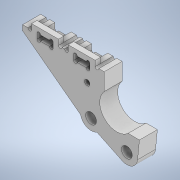
# Autodesk Inventor part: 後ろウィング固定フレーム中詰め
Saved by Autodesk Inventor 2020.2 (Build 242310000, 310)
## iProperties
Created: 2020-05-06
Part Number: 後ろウィング固定フレーム中詰め
Material: 一般
Document SubType Name: Modeling
Designer: mozar
Density: 1 g/cm^3
Appearance: 既定
Author: mozar
Autodesk Inventor part; units mm, degrees
ref_plane "YZ Plane" through (0, 0, 0) normal (1, 0, 0) x (0, 1, 0)
ref_plane "XZ Plane" through (0, 0, 0) normal (0, 1, 0) x (-1, 0, 0)
ref_plane "XY Plane" through (0, 0, 0) normal (0, 0, 1) x (1, 0, 0)
sketch "スケッチ1" plane through (0, 0, 0) normal (0, 0, 1) x (1, 0, 0)
  circle A0 centre (111.885, -19) radius 1.5
  line L0 (89.885, -6) -> (94.885, -6)
  arc A1 (94.885, -6) -> (96.885, -6) centre (95.885, -6) ccw
  line L1 (96.885, -6) -> (96.885, -3)
  arc A2 (96.885, -3) -> (94.885, -3) centre (95.885, -3) ccw
  line L2 (94.885, -3) -> (89.885, -3)
  arc A3 (89.885, -3) -> (87.885, -3) centre (88.885, -3) ccw
  line L3 (87.885, -3) -> (87.885, -6)
  arc A4 (87.885, -6) -> (89.885, -6) centre (88.885, -6) ccw
  arc A5 (76.4397, -3) -> (74.4397, -3) centre (75.4397, -3) ccw
  line L4 (74.4397, -3) -> (69.4397, -3)
  arc A6 (69.4397, -3) -> (67.4397, -3) centre (68.4397, -3) ccw
  line L5 (67.4397, -3) -> (67.4397, -6)
  arc A7 (67.4397, -6) -> (69.4397, -6) centre (68.4397, -6) ccw
  line L6 (69.4397, -6) -> (74.4397, -6)
  arc A8 (74.4397, -6) -> (76.4397, -6) centre (75.4397, -6) ccw
  line L7 (76.4397, -6) -> (76.4397, -3)
  line L8 (64.4397, -3) -> (64.4397, 0)
  line L9 (64.4397, 0) -> (79.4397, 0)
  line L10 (79.4397, 0) -> (79.4397, -3)
  arc A9 (79.4397, -3) -> (81.4397, -3) centre (80.4397, -3) ccw
  line L11 (81.4397, -3) -> (82.885, -3)
  arc A10 (82.885, -3) -> (84.885, -3) centre (83.885, -3) ccw
  line L12 (84.885, -3) -> (84.885, 0)
  line L13 (84.885, 0) -> (99.885, 0)
  line L14 (99.885, 0) -> (99.885, -3)
  arc A11 (99.885, -3) -> (101.885, -3) centre (100.885, -3) ccw
  line L15 (101.885, -3) -> (104.8897, -3)
  line L16 (104.8897, -3) -> (116.6369, -13.86)
  arc A12 (108.6424, -25.2037) -> (116.6369, -13.86) centre (111.885, -19) ccw
  arc A13 (108.5771, -25.2225) -> (108.6424, -25.2037) centre (95.0604, 21.7941) ccw
  line L17 (108.5771, -25.2225) -> (69.3788, -9.8882)
  arc A14 (65.1115, -8.2188) -> (69.3788, -9.8882) centre (68.4397, -6) ccw
  line L18 (65.1115, -8.2188) -> (59.4397, -6)
  line L19 (59.4397, -6) -> (59.4397, -3)
  line L20 (59.4397, -3) -> (62.4397, -3)
  arc A15 (62.4397, -3) -> (64.4397, -3) centre (63.4397, -3) ccw
  circle A16 centre (111.885, -19) radius 9
  circle A17 centre (111.885, -19) radius 9.5
  line L21 (111.8011, -25.9995) -> (171.7968, -26.719)
  circle A18 centre (111.885, -19) radius 14.5
  line L22 (111.7412, -30.9991) -> (171.7368, -31.7186)
  line L23 (93.2393, -9) -> (91.5308, -9)
  arc A19 (84.885, -6) -> (91.5308, -9) centre (88.885, -6) ccw
  line L24 (84.885, -6) -> (84.885, -3)
  arc A20 (91.5308, 0) -> (84.885, -3) centre (88.885, -3) ccw
  line L25 (91.5308, 0) -> (93.2393, 0)
  arc A21 (99.885, -3) -> (93.2393, 0) centre (95.885, -3) ccw
  line L26 (99.885, -3) -> (99.885, -6)
  arc A22 (93.2393, -9) -> (99.885, -6) centre (95.885, -6) ccw
  line L27 (72.7939, -9) -> (71.0854, -9)
  arc A23 (64.4397, -6) -> (71.0854, -9) centre (68.4397, -6) ccw
  line L28 (64.4397, -6) -> (64.4397, -3)
  arc A24 (71.0854, 0) -> (64.4397, -3) centre (68.4397, -3) ccw
  line L29 (71.0854, 0) -> (72.7939, 0)
  arc A25 (79.4397, -3) -> (72.7939, 0) centre (75.4397, -3) ccw
  line L30 (79.4397, -3) -> (79.4397, -6)
  arc A26 (72.7939, -9) -> (79.4397, -6) centre (75.4397, -6) ccw
  line L31 (69.2325, -6.6095) -> (108.7075, -22.0521)
  arc A27 (108.7075, -22.0521) -> (109.1445, -21.9137) centre (95.0604, 21.7941) ccw
  arc A28 (109.1445, -21.9137) -> (114.6004, -16.0628) centre (111.885, -19) ccw
  line L32 (114.6004, -16.0628) -> (103.7154, -6)
  line L33 (103.7154, -6) -> (103.5308, -6)
  arc A29 (96.885, -3) -> (103.5308, -6) centre (100.885, -3) ccw
  line L34 (96.885, -3) -> (87.885, -3)
  arc A30 (82.1624, -6.61) -> (87.885, -3) centre (83.885, -3) ccw
  arc A31 (76.4397, -3) -> (82.1624, -6.61) centre (80.4397, -3) ccw
  line L35 (76.4397, -3) -> (67.4397, -3)
  arc A32 (66.5221, -5.5493) -> (67.4397, -3) centre (63.4397, -3) ccw
  line L36 (66.5221, -5.5493) -> (67.4438, -5.9098)
  arc A33 (67.4438, -5.9098) -> (69.2325, -6.6095) centre (68.4397, -6) ccw
  circle A34 centre (111.885, -19) radius 1.5
  line L37 (111.885, -19) -> (111.885, 12.5174) construction
  line L38 (118.885, -19) -> (118.885, 12.5174)
  line L39 (104.885, 12.5174) -> (104.885, -19)
  arc A35 (104.885, -19) -> (118.885, -19) centre (111.885, -19) ccw
  arc A36 (118.885, 12.5174) -> (104.885, 12.5174) centre (111.885, 12.5174) ccw
  circle A37 centre (95.4507, -12.9865) radius 3
  circle A38 centre (121.1072, -35.6118) radius 4.5
  circle A39 centre (71.9397, -13.746) radius 4.5
  line L40 (118.9115, -39.5397) -> (104.8098, -31.6566)
  line L41 (106.4851, -32.457) -> (70.2638, -17.9223)
  line L42 (125.2948, -33.9642) -> (118.399, -16.4372)
  arc A40 (108.6424, -25.2037) -> (116.6369, -13.86) centre (111.885, -19) ccw
  point P0 (0, 0)
  point P1 (0, 0)
  point P2 (111.885, -3.2413)
  point P3 (69.5283, -9.9466)
  point P4 (118.885, -17.6725)
  point P5 (118.399, -16.4372)
  point P6 (123.0482, -28.2539)
  point P7 (105.6218, -32.1106)
  point P8 (97.5091, -20.8927)
  point P9 (107.3125, -5.2398)
  point P10 (104.885, -6.3016)
  point P11 (104.885, -3)
  dimension "d10" = 9
  dimension "d0" = 18
  dimension "d1" = 0.5
  dimension "d2" = 5
  dimension "d3" = 5
  dimension "d4" = 3
  dimension "d5" = 3
  dimension "d6" = 3
  dimension "d7" = 14
  dimension "d8" = 6
  dimension "d9" = 9
  constraints: 88 end point, 71 point on circle, 40 centre point, 13 tangent, 2 parallel, 1 coincident, 1 midpoint, 1 vertical, 33 other
  measures "d0" diameter of A16
  measures "d1" radial gap between concentric circles of A16 A17
  measures "d2" radial gap between concentric circles of A17 A18
  measures "d3" distance between parallel lines of L21 L22
  measures "d4" distance between parallel lines of L0 L23
  measures "d5" distance between parallel lines of L6 L27
  measures "d6" distance between parallel lines of L17 L31
  measures "d7" diameter of A36
  measures "d8" diameter of A37
  measures "d9" diameter of A38
sketch "スケッチ2" plane through (0, 0, 0) normal (0, 0, 1) x (1, 0, 0)
  circle A0 centre (111.885, -19) radius 9.5 projected
  circle A1 centre (111.885, -19) radius 14.5 projected
  circle A2 centre (117.5177, -35.5687) radius 4.5
  circle A3 centre (71.9397, -13.746) radius 4.5 projected
  circle A4 centre (95.4507, -12.9865) radius 3 projected
  arc A5 (96.885, -3) -> (103.5308, -6) centre (100.885, -3) ccw projected
  line L0 (101.885, -3) -> (104.8897, -3) projected
  line L1 (59.4397, -3) -> (62.4397, -3) projected
  line L2 (59.4397, -6) -> (59.4397, -3) projected
  arc A6 (94.885, -6) -> (96.885, -6) centre (95.885, -6) ccw projected
  line L3 (96.885, -6) -> (96.885, -3) projected
  arc A7 (96.885, -3) -> (94.885, -3) centre (95.885, -3) ccw projected
  arc A8 (89.885, -3) -> (87.885, -3) centre (88.885, -3) ccw projected
  line L4 (87.885, -3) -> (87.885, -6) projected
  arc A9 (87.885, -6) -> (89.885, -6) centre (88.885, -6) ccw projected
  line L5 (89.885, -6) -> (94.885, -6) projected
  line L6 (94.885, -3) -> (89.885, -3) projected
  arc A10 (76.4397, -3) -> (74.4397, -3) centre (75.4397, -3) ccw projected
  line L7 (74.4397, -3) -> (69.4397, -3) projected
  arc A11 (69.4397, -3) -> (67.4397, -3) centre (68.4397, -3) ccw projected
  line L8 (67.4397, -3) -> (67.4397, -6) projected
  arc A12 (67.4438, -5.9098) -> (69.2325, -6.6095) centre (68.4397, -6) ccw projected
  line L9 (69.4397, -6) -> (74.4397, -6) projected
  arc A13 (74.4397, -6) -> (76.4397, -6) centre (75.4397, -6) ccw projected
  line L10 (76.4397, -6) -> (76.4397, -3) projected
  line L11 (111.7412, -30.9991) -> (171.7368, -31.7186) projected
  line L12 (111.8011, -25.9995) -> (171.7968, -26.719) projected
  circle A14 centre (117.5177, -35.5687) radius 3
  circle A15 centre (71.9397, -13.746) radius 3
  circle A16 centre (117.5177, -35.5687) radius 6
  circle A17 centre (95.4507, -12.9865) radius 6
  circle A18 centre (71.9397, -13.746) radius 6
  line L13 (111.885, -19) -> (111.885, 24.2673) construction
  line L14 (118.885, -19) -> (118.885, 24.2673)
  line L15 (104.885, 24.2673) -> (104.885, -19)
  arc A19 (104.885, -19) -> (118.885, -19) centre (111.885, -19) ccw
  arc A20 (118.885, 24.2673) -> (104.885, 24.2673) centre (111.885, 24.2673) ccw
  line L16 (123.4874, -36.1712) -> (124.4986, -26.1518)
  line L17 (101.885, -3) -> (62.4397, -3)
  line L18 (59.4397, -6) -> (66.9734, -17.1128)
  line L19 (114.9266, -40.9804) -> (69.3486, -19.1576)
  arc A21 (69.2325, -6.6095) -> (69.4397, -6) centre (68.4397, -6) ccw
  point P0 (0, 0)
  point P1 (111.885, 2.6337)
  point P2 (118.2233, -26.0765)
  point P3 (104.885, -12.5774)
  point P4 (104.885, -3)
  point P5 (87.885, -3)
  point P6 (76.4397, -3)
  point P7 (67.4397, -3)
  dimension "d11" = 6
  dimension "d12" = 6
  dimension "d13" = 3
  dimension "d14" = 3
  dimension "d15" = 3
  dimension "d16" = 14
  dimension "d52" = 9
  constraints: 16 end point, 10 point on circle, 9 centre point, 9 tangent, 3 coincident, 1 horizontal, 1 midpoint, 1 parallel, 1 point on line, 1 vertical, 3 other
  measures "d11" diameter of A14
  measures "d12" diameter of A15
  measures "d13" radial gap between concentric circles of A14 A16
  measures "d14" radial gap between concentric circles of A4 A17
  measures "d15" radial gap between concentric circles of A15 A18
  measures "d16" diameter of A20
  measures "d52" diameter of A2
extrude "押し出し1" add sketch "スケッチ2" against normal blind 10 contours L12 A1 A16 A17 L15 A0 | L16 L11 A16 A1 | A1 A17 A6 L3 L17 L0 L15 | A16 L11 A1 | A1 L11 A16 | L16 A16 L11 | A17 A1 | A4 | A1 A17 | L11 A16 A1 A2 | A1 A2 L11 | L11 A2 A1 A16 | A17 A1 A16 L19 A18 L18 L2 L1 L17 L8 A12 A21 L9 A13 L10 L4 A9 L5 A6 | A14 | A2 A1 | A1 A2 | A18 | A3 | A15
hole "穴1" at (71.9397, -13.746, 0) at (95.4507, -12.9865, 0) at (117.5177, -35.5687, 0) direction (0, 0, -1) diameter 6 depth 12 tip angle 118
sketch "スケッチ3" plane through (0, 0, 0) normal (0, 0, 1) x (1, 0, 0)
  line L0 (-101.5, 48) -> (108.5, 48)
  circle A0 centre (111.885, -19) radius 4
  circle A1 centre (171.8807, -19.7195) radius 4
  circle A2 centre (111.885, -19) radius 7
  circle A3 centre (171.8807, -19.7195) radius 7
  line L1 (171.8807, -19.7195) -> (111.885, -19) construction
  line L2 (171.9647, -12.72) -> (111.969, -12.0005)
  line L3 (111.8011, -25.9995) -> (171.7968, -26.719)
  arc A4 (171.7968, -26.719) -> (171.9647, -12.72) centre (171.8807, -19.7195) ccw
  arc A5 (111.969, -12.0005) -> (111.8011, -25.9995) centre (111.885, -19) ccw
  line L4 (173.7961, -12.9866) -> (250.1906, -34.7195)
  circle A6 centre (241.9819, -63.5746) radius 30
  line L5 (268.18, -78.1916) -> (221.9512, -41.2414)
  line L6 (221.9512, -41.2414) -> (169.9654, -26.4523)
  line L7 (271.9819, -113.1361) -> (271.9819, -54.8199)
  line L8 (111.885, -19) -> (111.885, 41) construction
  line L9 (118.885, -19) -> (118.885, 41)
  line L10 (104.885, 41) -> (104.885, -19)
  arc A7 (104.885, -19) -> (118.885, -19) centre (111.885, -19) ccw
  arc A8 (118.885, 41) -> (104.885, 41) centre (111.885, 41) ccw
  circle A9 centre (29.4318, 47.238) radius 30
  line L11 (113.3193, 34.1485) -> (35.5787, 17.8745)
  line L12 (-0.5585, 48) -> (57.5489, 36.7771)
  line L13 (57.5489, 36.7771) -> (110.4508, 47.8515)
  circle A10 centre (113.5, -20) radius 68
  line L14 (321.9635, -82.9551) -> (60.2705, 100.2843)
  line L15 (259.1892, -39) -> (111.885, -19)
  arc A11 (93.5924, -27.1048) -> (135.371, -5.9244) centre (95.0604, 21.7941) ccw
  arc A12 (135.371, -5.9244) -> (135.8476, -3.6716) centre (132.899, -4.2246) ccw
  arc A13 (135.8476, -3.6716) -> (83.1833, 18.5565) centre (102.1579, -9.9896) ccw
  line L16 (111.885, -19) -> (112.6892, 40.9946) construction
  line L17 (118.8844, -19.0938) -> (119.6886, 40.9008)
  line L18 (105.6898, 41.0884) -> (104.8857, -18.9062)
  arc A14 (104.8857, -18.9062) -> (118.8844, -19.0938) centre (111.885, -19) ccw
  arc A15 (119.6886, 40.9008) -> (105.6898, 41.0884) centre (112.6892, 40.9946) ccw
  line L19 (164.9949, 48) -> (164.9949, 26)
  line L20 (164.9949, 26) -> (327.4949, -102)
  circle A16 centre (116.2926, -40) radius 68
  circle A17 centre (-98.885, 0) radius 67.5
  line L21 (321.3633, -8.501) -> (-152.6681, 78.4982)
  line L22 (104.8897, -3) -> (104.8897, 0)
  line L23 (104.8897, -3) -> (72.0656, -3)
  line L24 (72.0656, 0) -> (104.8897, 0)
  circle A18 centre (83.3769, -17.5) radius 13.85
  point P0 (0, 0)
  point P1 (141.8829, -19.3597)
  point P2 (111.885, 11)
  point P3 (105.885, 0)
  point P4 (105.885, 0)
  point P5 (23.7328, -42.729)
  point P6 (112.2871, 10.9973)
  dimension "d26" = 8
  dimension "d27" = 8
  dimension "d28" = 3
  dimension "d29" = 3
  dimension "d30" = 60
  dimension "d31" = 14
  dimension "d32" = 14
  dimension "d33" = 60
  dimension "d34" = 14
  dimension "d35" = 60
  dimension "d36" = 14
  dimension "d37" = 6
  dimension "d38" = 35
  dimension "d39" = 13.271
  dimension "d40" = 14
  dimension "d41" = 20
  dimension "d42" = 15
  dimension "d43" = 22
  dimension "d44" = 150
  dimension "d45" = 162.5
  dimension "d46" = 0
  dimension "d47" = 136
  dimension "d48" = 136
  dimension "d49" = 135
  dimension "d50" = 38.227
  dimension "d51" = 18
  constraints: 56 end point, 28 point on circle, 25 tangent, 18 centre point, 4 equal length, 3 coincident, 3 horizontal, 3 midpoint, 3 parallel, 3 vertical, 2 point on line, 1 concentric, 15 other
  measures "d26" diameter of A0
  measures "d27" diameter of A1
  measures "d28" radial gap between concentric circles of A0 A2
  measures "d30" distance of L1.start L1.end
  measures "d31" diameter of A5
  measures "d32" distance from line of L4 L5.end
  measures "d33" diameter of A6
  measures "d34" diameter of A8
  measures "d35" diameter of A9
  measures "d36" distance from line of L11 L12.end
  measures "d37" horizontal distance of L1.end point (105.885, 0)
  measures "d38" angle of L14 L0
  measures "d40" diameter of A15
  measures "d41" vertical distance of L15.start L1.end
  measures "d42" vertical distance of L1.start L4.end
  measures "d43" distance of L19.start L19.end
  measures "d44" vertical distance of L19.start L20.end
  measures "d45" distance from line of L19 L20.end
  measures "d46" distance from line of L19.start L0
  measures "d47" diameter of A10
  measures "d48" diameter of A16
  measures "d49" diameter of A17
  measures "d50" angle of L0 L20
  measures "d51" distance from line of L5.start L20
sketch "スケッチ4" plane through (0, 0, 0) normal (0, 0, 1) x (1, 0, 0)
  circle A0 centre (117.5177, -35.5687) radius 1.5
  circle A1 centre (95.4507, -12.9865) radius 1.5
  circle A2 centre (97.5945, -29.101) radius 1.5
  circle A3 centre (111.885, -19) radius 1.5
  line L0 (116.6369, -13.86) -> (104.8897, -3)
  line L1 (104.8897, -3) -> (101.885, -3)
  arc A4 (99.885, -3) -> (101.885, -3) centre (100.885, -3) ccw
  line L2 (99.885, -3) -> (99.885, 0)
  line L3 (99.885, 0) -> (84.885, 0)
  line L4 (84.885, 0) -> (84.885, -3)
  arc A5 (82.885, -3) -> (84.885, -3) centre (83.885, -3) ccw
  line L5 (82.885, -3) -> (81.4397, -3)
  arc A6 (79.4397, -3) -> (81.4397, -3) centre (80.4397, -3) ccw
  line L6 (79.4397, -3) -> (79.4397, 0)
  line L7 (79.4397, 0) -> (64.4397, 0)
  line L8 (64.4397, 0) -> (64.4397, -3)
  arc A7 (62.4397, -3) -> (64.4397, -3) centre (63.4397, -3) ccw
  line L9 (62.4397, -3) -> (59.4397, -3)
  line L10 (59.4397, -3) -> (59.4397, -6)
  line L11 (59.4397, -6) -> (65.1115, -8.2188)
  arc A8 (65.1115, -8.2188) -> (69.3788, -9.8882) centre (68.4397, -6) ccw
  line L12 (69.3788, -9.8882) -> (97.5091, -20.8927)
  arc A9 (97.5091, -20.8927) -> (98.5543, -24.7045) centre (111.885, -19) ccw
  arc A10 (98.5543, -24.7045) -> (97.6262, -33.6009) centre (97.5945, -29.101) ccw
  line L13 (97.6262, -33.6009) -> (107.1669, -33.5336)
  line L14 (107.1669, -33.5336) -> (114.849, -39.192)
  arc A11 (114.849, -39.192) -> (121.9415, -34.7438) centre (117.5177, -35.5687) ccw
  line L15 (121.9415, -34.7438) -> (118.7664, -17.7168)
  arc A12 (118.7664, -17.7168) -> (116.6369, -13.86) centre (111.885, -19) ccw
  line L16 (69.4397, -3) -> (74.4397, -3)
  arc A13 (76.4397, -3) -> (74.4397, -3) centre (75.4397, -3) ccw
  line L17 (76.4397, -3) -> (76.4397, -6)
  arc A14 (74.4397, -6) -> (76.4397, -6) centre (75.4397, -6) ccw
  line L18 (74.4397, -6) -> (69.4397, -6)
  arc A15 (67.4397, -6) -> (69.4397, -6) centre (68.4397, -6) ccw
  line L19 (67.4397, -6) -> (67.4397, -3)
  arc A16 (69.4397, -3) -> (67.4397, -3) centre (68.4397, -3) ccw
  arc A17 (94.885, -6) -> (96.885, -6) centre (95.885, -6) ccw
  line L20 (94.885, -6) -> (89.885, -6)
  arc A18 (87.885, -6) -> (89.885, -6) centre (88.885, -6) ccw
  line L21 (87.885, -6) -> (87.885, -3)
  arc A19 (89.885, -3) -> (87.885, -3) centre (88.885, -3) ccw
  line L22 (89.885, -3) -> (94.885, -3)
  arc A20 (96.885, -3) -> (94.885, -3) centre (95.885, -3) ccw
  line L23 (96.885, -3) -> (96.885, -6)
  circle A21 centre (95.4507, -12.9865) radius 3 projected
  circle A22 centre (71.9397, -13.746) radius 3 projected
  circle A23 centre (117.5177, -35.5687) radius 3 projected
  arc A24 (87.885, -6) -> (89.885, -6) centre (88.885, -6) ccw projected
  line L24 (87.885, -6) -> (87.885, -3) projected
  line L25 (87.885, -3) -> (76.4397, -3) projected
  line L26 (76.4397, -3) -> (76.4397, -6) projected
  arc A25 (74.4397, -6) -> (76.4397, -6) centre (75.4397, -6) ccw projected
  line L27 (74.4397, -6) -> (69.4397, -6) projected
  arc A26 (67.4397, -6) -> (69.4397, -6) centre (68.4397, -6) ccw projected
  line L28 (67.4397, -6) -> (67.4397, -3) projected
  line L29 (67.4397, -3) -> (59.4397, -3) projected
  line L30 (59.4397, -3) -> (59.4397, -6) projected
  line L31 (59.4397, -6) -> (66.9734, -17.1128) projected
  arc A27 (66.9734, -17.1128) -> (69.3486, -19.1576) centre (71.9397, -13.746) ccw projected
  line L32 (69.3486, -19.1576) -> (114.9266, -40.9804) projected
  arc A28 (114.9266, -40.9804) -> (123.4874, -36.1712) centre (117.5177, -35.5687) ccw projected
  line L33 (123.4874, -36.1712) -> (124.4986, -26.1518) projected
  line L34 (124.4986, -26.1518) -> (118.2233, -26.0765) projected
  arc A29 (104.885, -12.5774) -> (118.2233, -26.0765) centre (111.885, -19) ccw projected
  line L35 (104.885, -12.5774) -> (104.885, -3) projected
  line L36 (104.885, -3) -> (96.885, -3) projected
  line L37 (96.885, -3) -> (96.885, -6) projected
  arc A30 (94.885, -6) -> (96.885, -6) centre (95.885, -6) ccw projected
  line L38 (94.885, -6) -> (89.885, -6) projected
  point P0 (0, 0)
  point P1 (0, 0)
  point P2 (74.2011, -11.7746)
  point P3 (71.6162, -10.7635)
  point P4 (99.4867, -33.5878)
  point P5 (93.3734, -30.6607)
  constraints: 48 end point, 34 point on circle, 21 centre point, 9 horizontal, 9 vertical, 89 other
extrude "押し出し2" add sketch "スケッチ4" against normal blind 10 contours L13 A10 L32 | L12 A22 picked at (72.7177, -11.1035)
extrude "押し出し3" cut sketch "スケッチ4" against normal blind 10 contours L32 A27 L31 L11 A8 L12 A22 A9 A10
hole "穴2" at (97.5945, -29.101, 0) direction (0, 0, -1) diameter 3 depth 12 tip angle 118
extrude "押し出し4" add sketch "スケッチ4" against normal blind 10 contours A21
sketch "スケッチ5" plane through (0, 0, 0) normal (0, 0, 1) x (1, 0, 0)
  circle A0 centre (95.4507, -12.9865) radius 1.5 projected
  circle A1 centre (97.5945, -29.101) radius 1.5 projected
  arc A2 (98.5543, -24.7045) -> (97.6262, -33.6009) centre (97.5945, -29.101) ccw projected
  line L0 (97.6262, -33.6009) -> (99.4867, -33.5878) projected
  line L1 (99.4867, -33.5878) -> (114.9266, -40.9804) projected
  arc A3 (114.9266, -40.9804) -> (123.4874, -36.1712) centre (117.5177, -35.5687) ccw projected
  line L2 (123.4874, -36.1712) -> (124.4986, -26.1518) projected
  line L3 (124.4986, -26.1518) -> (118.2233, -26.0765) projected
  arc A4 (104.885, -12.5774) -> (118.2233, -26.0765) centre (111.885, -19) ccw projected
  line L4 (104.885, -12.5774) -> (104.885, -3) projected
  line L5 (104.885, -3) -> (96.885, -3) projected
  line L6 (96.885, -3) -> (96.885, -6) projected
  arc A5 (94.885, -6) -> (96.885, -6) centre (95.885, -6) ccw projected
  line L7 (94.885, -6) -> (89.885, -6) projected
  arc A6 (87.885, -6) -> (89.885, -6) centre (88.885, -6) ccw projected
  line L8 (87.885, -6) -> (87.885, -3) projected
  line L9 (87.885, -3) -> (76.4397, -3) projected
  line L10 (76.4397, -3) -> (76.4397, -6) projected
  arc A7 (74.4397, -6) -> (76.4397, -6) centre (75.4397, -6) ccw projected
  line L11 (74.4397, -6) -> (69.4397, -6) projected
  arc A8 (67.4397, -6) -> (69.4397, -6) centre (68.4397, -6) ccw projected
  line L12 (67.4397, -6) -> (67.4397, -3) projected
  line L13 (67.4397, -3) -> (59.4397, -3) projected
  line L14 (59.4397, -3) -> (59.4397, -6) projected
  line L15 (59.4397, -6) -> (65.1115, -8.2188) projected
  arc A9 (65.1115, -8.2188) -> (69.3788, -9.8882) centre (68.4397, -6) ccw projected
  line L16 (69.3788, -9.8882) -> (97.5091, -20.8927) projected
  arc A10 (97.5091, -20.8927) -> (98.5543, -24.7045) centre (111.885, -19) ccw projected
  line L17 (96.885, -3) -> (104.885, -3) projected
  line L18 (99.885, -3) -> (84.885, -3)
  line L19 (84.885, -3) -> (84.885, 0)
  line L20 (84.885, 0) -> (99.885, 0)
  line L21 (99.885, 0) -> (99.885, -3)
  line L22 (76.4397, -3) -> (87.885, -3) projected
  line L23 (79.4397, -3) -> (64.4397, -3)
  line L24 (64.4397, -3) -> (64.4397, 0)
  line L25 (64.4397, 0) -> (79.4397, 0)
  line L26 (79.4397, 0) -> (79.4397, -3)
  circle A11 centre (95.885, -3) radius 1
  circle A12 centre (88.885, -3) radius 1
  circle A13 centre (75.4397, -3) radius 1
  circle A14 centre (68.4397, -3) radius 1
  line L27 (96.885, -3) -> (96.885, -6) projected
  line L28 (87.885, -6) -> (87.885, -3) projected
  line L29 (67.4397, -6) -> (67.4397, -3) projected
  point P0 (0, 0)
  point P1 (69.4397, -3)
  point P2 (74.4397, -3)
  point P3 (89.885, -3)
  point P4 (94.885, -3)
  dimension "d66" = 15
  dimension "d67" = 3
  dimension "d68" = 15
  dimension "d69" = 3
  dimension "d70" = 3
  dimension "d71" = 3
  dimension "d72" = 2
  dimension "d73" = 2
  dimension "d74" = 2
  dimension "d75" = 2
  constraints: 16 end point, 6 point on line, 4 centre point, 4 parallel, 4 tangent, 2 horizontal, 2 perpendicular
  measures "d66" distance of L19.end L20.end
  measures "d67" distance of L18.end L19.end
  measures "d68" distance of L24.end L25.end
  measures "d69" distance of L23.end L24.end
  measures "d70" distance between parallel lines of L19 L8
  measures "d71" distance between parallel lines of L26 L10
  measures "d72" diameter of A11
  measures "d73" diameter of A12
  measures "d74" diameter of A13
  measures "d75" diameter of A14
extrude "押し出し5" add sketch "スケッチ5" against normal blind 3 contours L24 L25 L26 L9 A13 L23 A14 L13 | L5 A11 L18 A12 L9 L19 L20 L21
sketch "スケッチ6" plane through (0, 0, 0) normal (0, 0, 1) x (1, 0, 0)
  line L0 (64.4397, -3) -> (59.4397, -3) projected
  line L1 (59.4397, -3) -> (59.4397, -6) projected
  line L2 (59.4397, -6) -> (65.1115, -8.2188) projected
  arc A0 (65.1115, -8.2188) -> (69.3788, -9.8882) centre (68.4397, -6) ccw projected
  line L3 (69.3788, -9.8882) -> (97.5091, -20.8927) projected
  arc A1 (97.5091, -20.8927) -> (98.5543, -24.7045) centre (111.885, -19) ccw projected
  arc A2 (98.5543, -24.7045) -> (97.6262, -33.6009) centre (97.5945, -29.101) ccw projected
  line L4 (97.6262, -33.6009) -> (99.4867, -33.5878) projected
  line L5 (99.4867, -33.5878) -> (114.9266, -40.9804) projected
  arc A3 (114.9266, -40.9804) -> (123.4874, -36.1712) centre (117.5177, -35.5687) ccw projected
  line L6 (123.4874, -36.1712) -> (124.4986, -26.1518) projected
  line L7 (124.4986, -26.1518) -> (118.2233, -26.0765) projected
  arc A4 (104.885, -12.5774) -> (118.2233, -26.0765) centre (111.885, -19) ccw projected
  line L8 (104.885, -12.5774) -> (104.885, -3) projected
  line L9 (104.885, -3) -> (99.885, -3) projected
  line L10 (99.885, -3) -> (99.885, 0) projected
  line L11 (99.885, 0) -> (84.885, 0) projected
  line L12 (84.885, 0) -> (84.885, -3) projected
  line L13 (84.885, -3) -> (79.4397, -3) projected
  line L14 (79.4397, -3) -> (79.4397, 0) projected
  line L15 (79.4397, 0) -> (64.4397, 0) projected
  line L16 (64.4397, 0) -> (64.4397, -3) projected
  arc A5 (69.4397, -3) -> (67.4397, -3) centre (68.4397, -3) ccw projected
  line L17 (69.4397, -3) -> (74.4397, -3) projected
  arc A6 (76.4397, -3) -> (74.4397, -3) centre (75.4397, -3) ccw projected
  line L18 (76.4397, -3) -> (76.4397, -6) projected
  arc A7 (74.4397, -6) -> (76.4397, -6) centre (75.4397, -6) ccw projected
  line L19 (74.4397, -6) -> (69.4397, -6) projected
  arc A8 (67.4397, -6) -> (69.4397, -6) centre (68.4397, -6) ccw projected
  line L20 (67.4397, -6) -> (67.4397, -3) projected
  circle A9 centre (95.4507, -12.9865) radius 1.5 projected
  circle A10 centre (97.5945, -29.101) radius 1.5 projected
  arc A11 (89.885, -3) -> (87.885, -3) centre (88.885, -3) ccw projected
  line L21 (89.885, -3) -> (94.885, -3) projected
  arc A12 (96.885, -3) -> (94.885, -3) centre (95.885, -3) ccw projected
  line L22 (96.885, -3) -> (96.885, -6) projected
  arc A13 (94.885, -6) -> (96.885, -6) centre (95.885, -6) ccw projected
  line L23 (94.885, -6) -> (89.885, -6) projected
  arc A14 (87.885, -6) -> (89.885, -6) centre (88.885, -6) ccw projected
  line L24 (87.885, -6) -> (87.885, -3) projected
  line L25 (99.885, -3) -> (104.885, -3) projected
  circle A15 centre (100.885, -3) radius 1
  line L26 (79.4397, -3) -> (84.885, -3) projected
  circle A16 centre (83.885, -3) radius 1
  circle A17 centre (80.4397, -3) radius 1
  line L27 (59.4397, -3) -> (64.4397, -3) projected
  circle A18 centre (63.4397, -3) radius 1
  line L28 (99.885, -3) -> (99.885, 0) projected
  line L29 (84.885, 0) -> (84.885, -3) projected
  line L30 (79.4397, -3) -> (79.4397, 0) projected
  point P0 (0, 0)
  dimension "d78" = 2
  dimension "d79" = 2
  dimension "d80" = 2
  dimension "d81" = 2
  constraints: 4 centre point, 4 point on line, 4 tangent
  measures "d78" diameter of A15
  measures "d79" diameter of A16
  measures "d80" diameter of A17
  measures "d81" diameter of A18
extrude "押し出し6" cut sketch "スケッチ6" against normal blind 10 contours A18 L0 | L0 A18 | A17 L13 | L13 A17 | A16 L13 | L13 A16 | A15 L9 | L9 A15
sketch "スケッチ7" plane through (0, 0, 0) normal (0, 0, 1) x (1, 0, 0)
  arc A0 (79.4397, -3) -> (81.4397, -3) centre (80.4397, -3) ccw projected
  line L0 (79.4397, -3) -> (79.4397, 0) projected
  line L1 (79.4397, 0) -> (64.4397, 0) projected
  line L2 (64.4397, 0) -> (64.4397, -3) projected
  arc A1 (62.4397, -3) -> (64.4397, -3) centre (63.4397, -3) ccw projected
  line L3 (62.4397, -3) -> (59.4397, -3) projected
  line L4 (59.4397, -3) -> (59.4397, -6) projected
  line L5 (59.4397, -6) -> (65.1115, -8.2188) projected
  arc A2 (65.1115, -8.2188) -> (69.3788, -9.8882) centre (68.4397, -6) ccw projected
  line L6 (69.3788, -9.8882) -> (97.5091, -20.8927) projected
  arc A3 (97.5091, -20.8927) -> (98.5543, -24.7045) centre (111.885, -19) ccw projected
  arc A4 (98.5543, -24.7045) -> (97.6262, -33.6009) centre (97.5945, -29.101) ccw projected
  line L7 (97.6262, -33.6009) -> (99.4867, -33.5878) projected
  line L8 (99.4867, -33.5878) -> (114.9266, -40.9804) projected
  arc A5 (114.9266, -40.9804) -> (123.4874, -36.1712) centre (117.5177, -35.5687) ccw projected
  line L9 (123.4874, -36.1712) -> (124.4986, -26.1518) projected
  line L10 (124.4986, -26.1518) -> (118.2233, -26.0765) projected
  arc A6 (104.885, -12.5774) -> (118.2233, -26.0765) centre (111.885, -19) ccw projected
  line L11 (104.885, -12.5774) -> (104.885, -3) projected
  line L12 (104.885, -3) -> (101.885, -3) projected
  arc A7 (99.885, -3) -> (101.885, -3) centre (100.885, -3) ccw projected
  line L13 (99.885, -3) -> (99.885, 0) projected
  line L14 (99.885, 0) -> (84.885, 0) projected
  line L15 (84.885, 0) -> (84.885, -3) projected
  arc A8 (82.885, -3) -> (84.885, -3) centre (83.885, -3) ccw projected
  line L16 (82.885, -3) -> (81.4397, -3) projected
  arc A9 (69.4397, -3) -> (67.4397, -3) centre (68.4397, -3) ccw projected
  line L17 (69.4397, -3) -> (74.4397, -3) projected
  arc A10 (76.4397, -3) -> (74.4397, -3) centre (75.4397, -3) ccw projected
  line L18 (76.4397, -3) -> (76.4397, -6) projected
  arc A11 (74.4397, -6) -> (76.4397, -6) centre (75.4397, -6) ccw projected
  line L19 (74.4397, -6) -> (69.4397, -6) projected
  arc A12 (67.4397, -6) -> (69.4397, -6) centre (68.4397, -6) ccw projected
  line L20 (67.4397, -6) -> (67.4397, -3) projected
  circle A13 centre (95.4507, -12.9865) radius 1.5 projected
  circle A14 centre (97.5945, -29.101) radius 1.5 projected
  arc A15 (89.885, -3) -> (87.885, -3) centre (88.885, -3) ccw projected
  line L21 (89.885, -3) -> (94.885, -3) projected
  arc A16 (96.885, -3) -> (94.885, -3) centre (95.885, -3) ccw projected
  line L22 (96.885, -3) -> (96.885, -6) projected
  arc A17 (94.885, -6) -> (96.885, -6) centre (95.885, -6) ccw projected
  line L23 (94.885, -6) -> (89.885, -6) projected
  arc A18 (87.885, -6) -> (89.885, -6) centre (88.885, -6) ccw projected
  line L24 (87.885, -6) -> (87.885, -3) projected
  arc A19 (98.5543, -24.7045) -> (97.6262, -33.6009) centre (97.5945, -29.101) ccw projected
  line L25 (59.4397, -3) -> (59.4397, -6) projected
  line L26 (94.8874, -32.6956) -> (59.4397, -6)
  arc A20 (98.5543, -24.7045) -> (97.6262, -33.6009) centre (97.5945, -29.101) ccw projected
  point P0 (0, 0)
  constraints: 2 end point, 1 point on circle, 1 tangent
extrude "押し出し7" add sketch "スケッチ7" against normal blind 10 contours L5 A2 L6 A3 A4 L26
sketch "スケッチ8" plane through (0, 0, 0) normal (0, 0, 1) x (1, 0, 0)
  arc A0 (79.4397, -3) -> (81.4397, -3) centre (80.4397, -3) ccw projected
  line L0 (79.4397, -3) -> (79.4397, 0) projected
  line L1 (79.4397, 0) -> (64.4397, 0) projected
  line L2 (64.4397, 0) -> (64.4397, -3) projected
  arc A1 (62.4397, -3) -> (64.4397, -3) centre (63.4397, -3) ccw projected
  line L3 (62.4397, -3) -> (59.4397, -3) projected
  line L4 (59.4397, -3) -> (59.4397, -6) projected
  line L5 (59.4397, -6) -> (94.8874, -32.6956) projected
  arc A2 (94.8874, -32.6956) -> (97.6262, -33.6009) centre (97.5945, -29.101) ccw projected
  line L6 (97.6262, -33.6009) -> (99.4867, -33.5878) projected
  line L7 (99.4867, -33.5878) -> (114.9266, -40.9804) projected
  arc A3 (114.9266, -40.9804) -> (123.4874, -36.1712) centre (117.5177, -35.5687) ccw projected
  line L8 (123.4874, -36.1712) -> (124.4986, -26.1518) projected
  line L9 (124.4986, -26.1518) -> (118.2233, -26.0765) projected
  arc A4 (104.885, -12.5774) -> (118.2233, -26.0765) centre (111.885, -19) ccw projected
  line L10 (104.885, -12.5774) -> (104.885, -3) projected
  line L11 (104.885, -3) -> (101.885, -3) projected
  arc A5 (99.885, -3) -> (101.885, -3) centre (100.885, -3) ccw projected
  line L12 (99.885, -3) -> (99.885, 0) projected
  line L13 (99.885, 0) -> (84.885, 0) projected
  line L14 (84.885, 0) -> (84.885, -3) projected
  arc A6 (82.885, -3) -> (84.885, -3) centre (83.885, -3) ccw projected
  line L15 (82.885, -3) -> (81.4397, -3) projected
  arc A7 (69.4397, -3) -> (67.4397, -3) centre (68.4397, -3) ccw projected
  line L16 (69.4397, -3) -> (74.4397, -3) projected
  arc A8 (76.4397, -3) -> (74.4397, -3) centre (75.4397, -3) ccw projected
  line L17 (76.4397, -3) -> (76.4397, -6) projected
  arc A9 (74.4397, -6) -> (76.4397, -6) centre (75.4397, -6) ccw projected
  line L18 (74.4397, -6) -> (69.4397, -6) projected
  arc A10 (67.4397, -6) -> (69.4397, -6) centre (68.4397, -6) ccw projected
  line L19 (67.4397, -6) -> (67.4397, -3) projected
  circle A11 centre (95.4507, -12.9865) radius 1.5 projected
  circle A12 centre (97.5945, -29.101) radius 1.5 projected
  arc A13 (89.885, -3) -> (87.885, -3) centre (88.885, -3) ccw projected
  line L20 (89.885, -3) -> (94.885, -3) projected
  arc A14 (96.885, -3) -> (94.885, -3) centre (95.885, -3) ccw projected
  line L21 (96.885, -3) -> (96.885, -6) projected
  arc A15 (94.885, -6) -> (96.885, -6) centre (95.885, -6) ccw projected
  line L22 (94.885, -6) -> (89.885, -6) projected
  arc A16 (87.885, -6) -> (89.885, -6) centre (88.885, -6) ccw projected
  line L23 (87.885, -6) -> (87.885, -3) projected
  circle A17 centre (117.5177, -35.5687) radius 3 projected
  circle A18 centre (97.5945, -29.101) radius 3
  circle A19 centre (97.5945, -29.101) radius 6
  point P0 (0, 0)
  point P1 (91.7172, -30.3082)
  point P2 (100.7605, -34.1977)
  dimension "d86" = 6
  dimension "d87" = 3
  constraints: 2 centre point, 1 coincident
  measures "d86" diameter of A18
  measures "d87" radial gap between concentric circles of A18 A19
extrude "押し出し8" add sketch "スケッチ8" against normal blind 10 contours L5 A2 L6 L7 A19 picked at (92.9262, -31.559)
extrude "押し出し9" cut sketch "スケッチ8" against normal blind 10 contours A12 | A18
equation "\"d35\" = d33"
equation "\"d71\" = d70"
